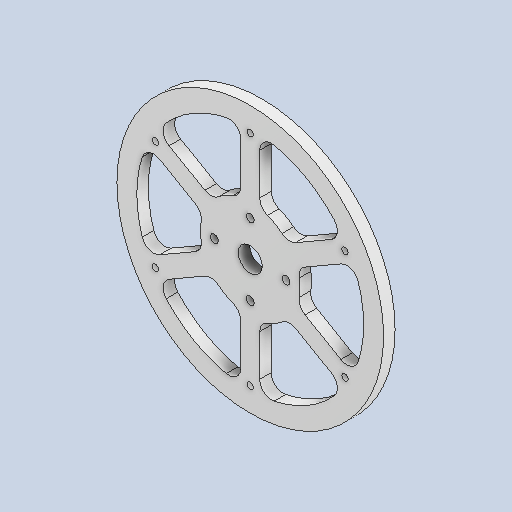
# Autodesk Inventor part: TH22_POM_roller_sn
Saved by Autodesk Inventor 2025.1 (Build 291241000, 241)
## iProperties
Created: 2021-11-15
Part Number: TH22_POM_roller_sn
Material: ABS プラスチック
Document SubType Name: Modeling
Designer: 中島 青蔵
Density: 1.06 g/cm^3
Appearance: 滑らか - 白
Author: 中島 青蔵
Autodesk Inventor part; units mm, degrees
ref_plane "YZ Plane" through (0, 0, 0) normal (1, 0, 0) x (0, 1, 0)
ref_plane "XZ Plane" through (0, 0, 0) normal (0, 1, 0) x (-1, 0, 0)
ref_plane "XY Plane" through (0, 0, 0) normal (0, 0, 1) x (1, 0, 0)
sketch "スケッチ1" plane through (0, 0, 0) normal (0, 0, 1) x (1, 0, 0)
  circle A0 centre (0, 0) radius 67
  circle A1 centre (0, 0) radius 57
  circle A2 centre (0, 0) radius 25
  line L0 (0, 0) -> (0, 67)
  circle A3 centre (0, 0) radius 6.05
  line L1 (4.7669, 0.7625) -> (4.7669, 66.8302)
  line L2 (4.7669, 0.7625) -> (70.8346, 0.7625) construction
  line L3 (-4.7669, 0.7625) -> (-4.7669, 66.8302)
  line L4 (-3.0438, -3.747) -> (-60.2601, 29.2869)
  line L5 (1.7231, 4.5095) -> (-55.4932, 37.5433)
  line L6 (1.7231, -4.5095) -> (-55.4932, -37.5433)
  line L7 (-3.0438, 3.747) -> (-60.2601, -29.2869)
  line L8 (4.7669, -0.7625) -> (4.7669, -66.8302)
  line L9 (-4.7669, -0.7625) -> (-4.7669, -66.8302)
  line L10 (3.0438, 3.747) -> (60.2601, -29.2869)
  line L11 (-1.7231, -4.5095) -> (55.4932, -37.5433)
  line L12 (-1.7231, 4.5095) -> (55.4932, 37.5433)
  line L13 (3.0438, -3.747) -> (60.2601, 29.2869)
  point P0 (4.7669, 56.8003)
  point P1 (46.8071, 32.5284)
  point P2 (18.87, 16.3989)
  point P3 (4.7669, 24.5413)
  point P4 (-4.7669, 56.8003)
  point P5 (-4.7669, 24.5413)
  point P6 (-18.87, 16.3989)
  point P7 (-46.8071, 32.5284)
  point P8 (51.574, -24.2719)
  point P9 (23.6368, -8.1424)
  point P10 (23.6368, 8.1424)
  point P11 (51.574, 24.2719)
  point P12 (4.7669, -56.8003)
  point P13 (4.7669, -24.5413)
  point P14 (18.87, -16.3989)
  point P15 (46.8071, -32.5284)
  point P16 (-46.8071, -32.5284)
  point P17 (-18.87, -16.3989)
  point P18 (-4.7669, -24.5413)
  point P19 (-4.7669, -56.8003)
  point P20 (-51.574, 24.2719)
  point P21 (-23.6368, 8.1424)
  point P22 (-23.6368, -8.1424)
  point P23 (-51.574, -24.2719)
  dimension "d0" = 134
  dimension "d1" = 114
  dimension "d2" = 50
  dimension "d3" = 12.1
  dimension "d4" = 90
  dimension "d7" = 360
  constraints: 28 end point, 4 centre point, 4 coincident, 2 point on circle, 2 symmetric about line, 1 horizontal, 1 perpendicular, 37 other
  measures "d0" diameter of A0
  measures "d1" diameter of A1
  measures "d2" diameter of A2
  measures "d3" diameter of A3
  measures "d4" angle of L2 L1
extrude "押し出し1" add sketch "スケッチ1" along normal blind 5.8 contours A0 L10 A1 L13 | L13 A1 L12 A0 | A0 L11 A1 L10 | L12 A1 L1 A0 | L13 A2 L12 A1 | A0 L8 A1 L11 | A1 L11 A2 L10 | L1 A1 L0 A0 | L13 L10 A3 L1 L12 A2 | A2 L10 L13 | A0 L9 A1 L8 | A2 L11 L8 A3 L13 L10 | L0 A1 L3 A0 | L1 A2 L0 A1 | L12 L1 A2 | L13 A3 L10 | A0 L6 A1 L9 | A1 L9 A2 L8 | A2 L8 L11 | L3 A1 L5 A0 | L0 A2 L3 A1 | L1 L12 A3 L0 A2 | L1 A3 L12 | A0 L7 A1 L6 | A2 L9 L6 A3 L11 L8 | L11 A3 L8 | L5 A1 L4 A0 | L0 A3 L5 L3 A2 | A0 L4 A1 L7 | A1 L7 A2 L6 | A2 L6 L9 | L5 A2 L4 A1 | L3 L5 A2 | A2 L7 L4 A3 L9 L6 | L9 A3 L6 | L5 L3 A3 L7 L4 A2 | L5 A3 L3 | A2 L4 L7 | L7 A3 L4
sketch "スケッチ2" plane through (0, 0, 5.8) normal (0, 0, 1) x (1, 0, 0)
  point P0 (0, 0)
  point P1 (0, 18)
  point P2 (-18, 0)
  point P3 (0, -18)
  point P4 (18, 0)
  point P5 (0, 55)
  point P6 (-47.6314, 27.5)
  point P7 (-47.6314, -27.5)
  point P8 (0, -55)
  point P9 (47.6314, -27.5)
  point P10 (47.6314, 27.5)
  dimension "d11" = 18
  dimension "d14" = 360
  dimension "d16" = 55
  dimension "d19" = 360
  constraints: 12 other
  measures "d11" distance of point (0, 0) point (0, 18)
  measures "d16" distance of point (0, 0) point (0, 55)
hole "穴1" at (0, 18, 5.8) at (-18, 0, 5.8) at (0, -18, 5.8) at (18, 0, 5.8) direction (0, 0, -1) diameter 4 end through all
hole "穴2" at (0, 55, 5.8) at (-47.6314, 27.5, 5.8) at (-47.6314, -27.5, 5.8) at (0, -55, 5.8) at (47.6314, -27.5, 5.8) at (47.6314, 27.5, 5.8) direction (0, 0, -1) diameter 3.2 end through all
fillet "フィレット1" radius 6 24 edges at (-51.574, 24.2719, 2.9) (-51.574, -24.2719, 2.9) (-23.6368, -8.1424, 2.9) (-23.6368, 8.1424, 2.9) (-46.8071, 32.5284, 2.9) (-18.87, 16.3989, 2.9) (-4.7669, 24.5413, 2.9) (-4.7669, 56.8003, 2.9) (4.7669, 56.8003, 2.9) (4.7669, 24.5413, 2.9) (18.87, 16.3989, 2.9) (46.8071, 32.5284, 2.9) (51.574, 24.2719, 2.9) (23.6368, 8.1424, 2.9) (23.6368, -8.1424, 2.9) (51.574, -24.2719, 2.9) (46.8071, -32.5284, 2.9) (18.87, -16.3989, 2.9) (4.7669, -24.5413, 2.9) (4.7669, -56.8003, 2.9) (-4.7669, -56.8003, 2.9) (-4.7669, -24.5413, 2.9) (-18.87, -16.3989, 2.9) (-46.8071, -32.5284, 2.9)
